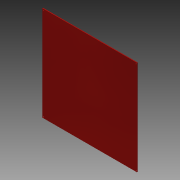
# Autodesk Inventor part: Heatbed
Saved by Autodesk Inventor 2014 (Build 180170000, 170)
## iProperties
Created: 2013-12-13
Part Number: Heatbed
Material: Aluminum, Anodized Red
Document SubType Name: Modeling
Designer: Bram
Density: 2.71 g/cm^3
Appearance: Anodized - Red
Author: Bram
Autodesk Inventor part; units mm, degrees
ref_plane "YZ Plane" through (0, 0, 0) normal (1, 0, 0) x (0, 1, 0)
ref_plane "XZ Plane" through (0, 0, 0) normal (0, 1, 0) x (-1, 0, 0)
ref_plane "XY Plane" through (0, 0, 0) normal (0, 0, 1) x (1, 0, 0)
sketch "Sketch1" plane through (0, 0, 0) normal (0, 1, 0) x (-1, 0, 0)
  line L0 (-107, 107) -> (107, 107)
  line L1 (107, 107) -> (107, -107)
  line L2 (107, -107) -> (-107, -107)
  line L3 (-107, -107) -> (-107, 107)
  line L4 (-107, 107) -> (107, -107) construction
  line L5 (107, 107) -> (-107, -107) construction
  point P0 (0, 0)
  dimension "d0" = 214
  dimension "d1" = 214
  constraints: 12 end point, 2 midpoint, 2 parallel, 1 horizontal, 1 perpendicular
  measures "d0" distance of L1.end L2.end
  measures "d1" distance of L0.end L1.end
extrude "Extrusion1" add sketch "Sketch1" along normal blind 1.6
sketch "Sketch2" plane through (0, 1.6, 0) normal (0, 1, 0) x (1, 0, 0)
  line L0 (-107, 107) -> (-107, -107) projected
  line L1 (0, 13.9914) -> (-10, -3.3291)
  line L2 (0, 13.9914) -> (20, 13.9914) construction
  line L3 (-10, -3.3291) -> (10, -3.3291)
  line L4 (10, -3.3291) -> (0, 13.9914)
  line L5 (-5.4032, 2.7326) -> (4.9323, 2.7326) construction
  line L6 (4.9323, 2.7326) -> (4.9323, -0.9149) construction
  line L7 (4.9323, -0.9149) -> (-5.4032, -0.9149) construction
  line L8 (-5.4032, -0.9149) -> (-5.4032, 2.7326) construction
  line L9 (0.0715, 16.0255) -> (-12.0985, -5.0535)
  line L10 (-12.0985, -5.0535) -> (12.2415, -5.0535)
  line L11 (12.2415, -5.0535) -> (0.0715, 16.0255)
  point P0 (0, 0)
  dimension "d4" = 20
  dimension "d6" = 20
  dimension "d9" = 24.34
  dimension "d10" = 24.34
  constraints: 14 end point, 1 equal length, 1 horizontal, 1 perpendicular, 2 other
  measures "d4" distance of L1.start L1.end
  measures "d6" distance of L1.end L3.end
  measures "d9" distance of L11.end L9.end
  measures "d10" distance of L9.end L11.start
extrude "Extrusion2" add sketch "Sketch2" along normal blind 0.1
sketch "Sketch3" plane through (0, 1.6, 0) normal (0, 1, 0) x (1, 0, 0)
  line L0 (104.5, -104.5) -> (-104.5, 104.5) construction
  circle A0 centre (-104.5, 104.5) radius 1.5
  circle A1 centre (104.5, 104.5) radius 1.5
  circle A2 centre (104.5, -104.5) radius 1.5
  circle A3 centre (-104.5, -104.5) radius 1.5
  point P0 (0, 0)
  dimension "d15" = 3
  dimension "d16" = 3
  dimension "d17" = 3
  dimension "d18" = 3
  constraints: 4 centre point, 2 coincident, 2 end point, 1 midpoint
  measures "d15" diameter of A0
  measures "d16" diameter of A1
  measures "d17" diameter of A2
  measures "d18" diameter of A3
extrude "Extrusion3" cut sketch "Sketch3" against normal blind 10
body "Solid1"
